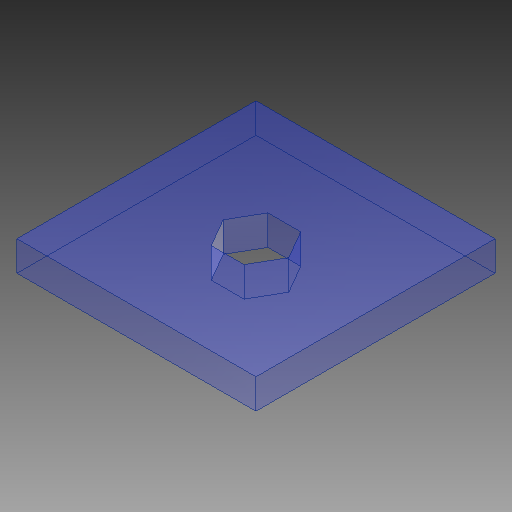
# Autodesk Inventor part: platform nut holder
Saved by Autodesk Inventor 2018.1 (Build 221171000, 171)
## iProperties
Created: 2017-07-29
Part Number: platform nut holder
Material: PVC-Piping
Document SubType Name: Modeling
Designer: Tom
Density: 1.4 g/cm^3
Appearance: Clear - Blue
Mass: 85.2231 g
Surface Area: 160.329 cm^2
Volume: 60.8736 cm^3
Author: Tom
Autodesk Inventor part; units mm, degrees
ref_plane "YZ Plane" through (0, 0, 0) normal (1, 0, 0) x (0, 1, 0)
ref_plane "XZ Plane" through (0, 0, 0) normal (0, 1, 0) x (-1, 0, 0)
ref_plane "XY Plane" through (0, 0, 0) normal (0, 0, 1) x (1, 0, 0)
sketch "Sketch1" plane through (0, 0, 0) normal (0, 0, 1) x (1, 0, 0)
  line L0 (0, 0) -> (80, 0)
  line L1 (80, 0) -> (80, 80)
  line L2 (80, 80) -> (0, 80)
  line L3 (0, 80) -> (0, 0)
  dimension "d4" = 80
  dimension "d5" = 80
  constraints: 8 end point, 2 parallel, 1 horizontal, 1 perpendicular
  measures "d4" distance of L1.end L2.end
  measures "d5" distance of L0.end L1.end
extrude "Extrusion1" add sketch "Sketch1" along normal blind 10
sketch "Sketch2" plane through (0, 0, 0) normal (0, 0, -1) x (-1, 0, 0)
  line L0 (-49.5, 34.5152) -> (-49.5, 45.4848) projected
  line L1 (-49.5, 45.4848) -> (-40, 50.9697) projected
  line L2 (-40, 50.9697) -> (-30.5, 45.4848) projected
  line L3 (-30.5, 45.4848) -> (-30.5, 34.5152) projected
  line L4 (-30.5, 34.5152) -> (-40, 29.0303) projected
  line L5 (-40, 29.0303) -> (-49.5, 34.5152) projected
  point P0 (0, 0)
extrude "Extrusion2" cut sketch "Sketch2" against normal blind 20
equation "\"d4\" = 2 * nutdist"
equation "\"d5\" = 2 * nutdist"
equation "\"d0\" = nutholdert"
equation "\"d2\" = platft"
equation "\"lcsd\" = 19.05"
equation "\"lcwd1\" = 25"
equation "\"lcwd2\" = 34"
equation "\"lch1\" = 39"
equation "\"lcwd3\" = 43"
equation "\"dia1\" = 6"
equation "\"td\" = 18"
equation "\"bhh\" = 6"
equation "\"sw\" = 25"
equation "\"sh\" = 31"
equation "\"spacert\" = 2"
equation "\"platft\" = 20"
equation "\"pvct\" = 5"
equation "\"dia3\" = 8"
equation "\"dia4\" = 11"
equation "\"tankl\" = 379"
equation "\"play\" = 9"
equation "\"holeh\" = 26"
equation "\"surroundt\" = 5"
equation "\"slack\" = 0.5"
equation "\"play2\" = 3"
equation "\"diawater\" = 25"
equation "\"diaoverflow\" = 25"
equation "\"diaph\" = 32"
equation "\"diacucl\" = 32"
equation "\"diaair\" = 32"
equation "\"diasurroundhole\" = 42"
equation "\"diagrate\" = 12"
equation "\"gratespacing\" = 12.02082"
equation "\"sidedist\" = 13.9375"
equation "\"bottomdist\" = 9.6355"
equation "\"diahcl\" = 32"
equation "\"bracketwtop\" = 6"
equation "\"bracketwbottom\" = 6"
equation "\"nett\" = 1"
equation "\"nethole\" = 16"
equation "\"netside\" = 3.5"
equation "\"nettop\" = 7"
equation "\"netholespacing\" = 2"
equation "\"nutholdert\" = 10"
equation "\"diaetape\" = 32"
equation "\"nutdist\" = 40"
body "Solid1"
